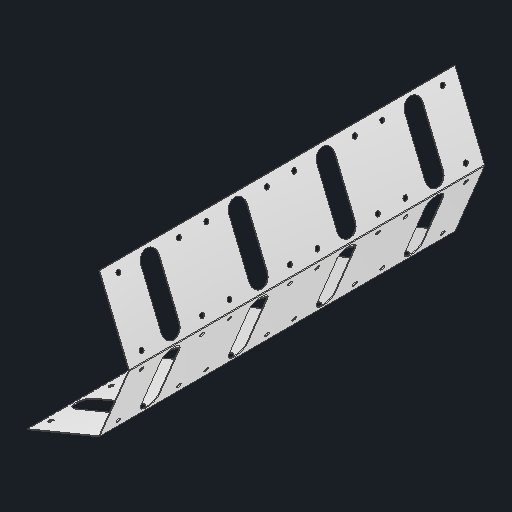
# Autodesk Inventor part: DMF 01 14 Барабан Лист прав брт v2.1
Saved by Autodesk Inventor 2026.2 (Build 302298000, 298)
## iProperties
Created: 2024-04-28
Part Number: DMF 01 14 Барабан Лист прав брт v2.1
Material: Stainless Steel AISI 304
Document SubType Name: Sheet Metal
Designer: pokla
Density: 8 g/cm^3
Appearance: Chrome - Satin
Sheet Metal Rule: Default
Flat Pattern Width: 63.6056 cm
Flat Pattern Length: 97 cm
Flat Pattern Area: 6169.75 cm^2
Sheet Metal Width: 636,056 mm
Sheet Metal Length: 970,000 mm
Sheet Metal Area: 616974,737 mm^2
Stock Number: Барабан_Лист_Правый_Борт
d174: 145,000 mm
d175: 50,000 mm
Author: pokla
Autodesk Inventor part; units mm, degrees
ref_plane "YZ Plane" through (0, 0, 0) normal (1, 0, 0) x (0, 1, 0)
ref_plane "XZ Plane" through (0, 0, 0) normal (0, 1, 0) x (-1, 0, 0)
ref_plane "XY Plane" through (0, 0, 0) normal (0, 0, 1) x (1, 0, 0)
sketch "Sketch2" plane through (0, 0, 0) normal (0, 0, 1) x (1, 0, 0)
  line L0 (0, 278.715992) -> (197.081968, 197.081968) construction
  line L1 (197.081968, 197.081968) -> (278.715992, 0) construction
  line L2 (278.715992, 0) -> (197.081968, -197.081968) construction
  line L3 (197.081968, -197.081968) -> (0, -278.715992) construction
  line L4 (0, -278.715992) -> (-197.081968, -197.081968) construction
  line L5 (-197.081968, -197.081968) -> (-278.715992, 0) construction
  line L6 (-278.715992, 0) -> (-197.081968, 197.081968) construction
  line L7 (-197.081968, 197.081968) -> (0, 278.715992) construction
  line L8 (197.426383, 196.250476) -> (278.081941, 1.530734)
  line L9 (278.081941, -1.530734) -> (197.716018, -195.551234)
  arc A0 (278.081941, -1.530734) -> (278.081941, 1.530734) centre (274.386423, 0) ccw
  line L10 (195.551234, -197.716018) -> (0.831492, -278.371576)
  arc A1 (195.551234, -197.716018) -> (197.716018, -195.551234) centre (194.0205, -194.0205) ccw
  line L11 (278.715992, 0) -> (278.081941, 1.530734) construction
  line L12 (278.081941, 1.530734) -> (279.612675, 2.164784) construction
  line L13 (279.612675, 2.164784) -> (280.246725, 0.634051) construction
  line L14 (280.246725, 0.634051) -> (278.715992, 0) construction
  line L15 (1.530734, 278.081941) -> (0, 278.715992) construction
  line L16 (0, 278.715992) -> (0.634051, 280.246725) construction
  line L17 (0.634051, 280.246725) -> (2.164784, 279.612675) construction
  line L18 (2.164784, 279.612675) -> (1.530734, 278.081941) construction
  point P0 (0, 0)
  point P1 (0, 0)
  dimension "d56" = 515
  dimension "d58" = 4
  dimension "d69" = 0.9
  dimension "d70" = 4
  dimension "d149" = 0.9
  measures "d56" distance between parallel lines of L6 L2
  measures "d58" radius of A0
  measures "d69" distance of L3.end L10.end
  measures "d70" radius of A1
  measures "d149" distance of L0.end L8.start
contour flange "Contour Flange2" sketch "Sketch2" thickness 2 bend radius 2 width 970 along (0, 0, 1) mid plane no both sides no wall seen from (237.754162, 98.890605, 0) lies toward (-0.9238795, -0.3826834, 0) curves L8 A0 L9 A1 L10
bend "Bend2"
corner "Corner2"
sketch "Sketch13" plane through (197.716018, -195.551234, 970) normal (0.9238795, -0.3826834, 0) x (0, 0, -1)
  line L0 (0, 0) -> (0, 210.006276)
  line L1 (970, 210.006276) -> (970, 0)
  line L2 (820, 177.503138) -> (870, 177.503138) construction
  line L3 (870, 177.503138) -> (870, 32.503138)
  line L4 (870, 32.503138) -> (820, 32.503138) construction
  line L5 (820, 32.503138) -> (820, 177.503138)
  line L6 (820, 177.503138) -> (870, 32.503138) construction
  line L7 (870, 177.503138) -> (820, 32.503138) construction
  arc A0 (870, 177.503138) -> (820, 177.503138) centre (845, 177.503138) ccw
  arc A1 (820, 32.503138) -> (870, 32.503138) centre (845, 32.503138) ccw
  circle A2 centre (762.5, 187.503138) radius 5.5 construction
  circle A3 centre (927.5, 187.503138) radius 5.5 construction
  line L8 (845, 177.503138) -> (845, 32.503138) construction
  line L9 (870, 105.003138) -> (820, 105.003138) construction
  circle A4 centre (762.5, 22.503138) radius 5.5 construction
  circle A5 centre (927.5, 22.503138) radius 5.5 construction
  circle A6 centre (762.5, 187.503138) radius 6.5
  circle A7 centre (845, 187.503138) radius 6.5 construction
  circle A8 centre (845, 22.503138) radius 6.5 construction
  circle A9 centre (762.5, 22.503138) radius 6.5
  circle A10 centre (927.5, 22.503138) radius 6.5
  circle A11 centre (927.5, 187.503138) radius 6.5
  point P0 (970, 105.003138)
  point P1 (0, 105.003138)
  point P2 (845, 105.003138)
  point P3 (845, 105.003138)
  point P4 (970, 105.003138)
  dimension "d166" = 145
  dimension "d167" = 50
  dimension "d168" = 165
  dimension "d169" = 165
  dimension "d170" = 11
  dimension "d171" = 13
  dimension "d172" = 13
  dimension "d173" = 165
  dimension "d176" = 100
  constraints: 16 end point, 12 centre point, 7 midpoint, 4 coincident, 4 point on circle, 4 tangent, 3 equal radius, 2 parallel, 2 point on line, 1 horizontal, 1 horizontal alignment, 1 perpendicular, 1 vertical, 4 other
  measures "d166" distance of L2.end L3.end
  measures "d167" distance of L2.start L2.end
  measures "d168" distance of A3.centre A2.centre
  measures "d169" distance of A5.centre A3.centre
  measures "d170" diameter of A2
  measures "d171" diameter of A6
  measures "d172" diameter of A7
  measures "d173" distance of A8.centre A7.centre
  measures "d176" distance between parallel lines of L1 L3
extrude "Cut2" cut sketch "Sketch13" against normal blind 2
pattern_linear "Rectangular Pattern4" count 4 spacing 240 along (0, 0, 1) of "Cut2"
pattern_circular "Circular Pattern3" count 3 over 90 about axis through (0, 0, -10) along (0, 0, 1) of "Cut2", "Rectangular Pattern4" both ways yes
equation "\"d56\" = Барабан_размер_по_плоскостям"
equation "\"d58\" = BendRadius + Thickness"
equation "\"d69\" = Барабан_отступ_развертки"
equation "\"d70\" = BendRadius + Thickness"
equation "\"d25\" = Thickness"
equation "\"d26\" = BendReliefWidth"
equation "\"d27\" = BendReliefDepth"
equation "\"d28\" = MinimumRemnant"
equation "\"d29\" = TransitionRadius"
equation "\"d31\" = BendRadius"
equation "\"d33\" = CornerReliefSize"
equation "\"d34\" = GapSize"
equation "\"d35\" = JacobiRadiusSize"
equation "\"BendRadius\" = Thickness"
equation "\"BendReliefWidth\" = Thickness"
equation "\"BendReliefDepth\" = 0.5 * Thickness"
equation "\"CornerReliefSize\" = 4 * Thickness"
equation "\"MinimumRemnant\" = 2 * Thickness"
equation "\"TransitionRadius\" = BendRadius"
equation "\"JacobiRadiusSize\" = BendRadius"
equation "\"GapSize\" = Thickness"
equation "\"d174\" = 145"
equation "\"Барабан_размер_по_плоскостям\" = 515"
equation "\"Thickness\" = 2"
equation "\"Барабан_отступ_развертки\" = 0.9"
body "Solid2"
